Autodesk Inventor part; units mm, degrees
(part 2 of 2)
  spline S117 degree 2 poles (-26.5872, -18.3544) (-26.5872, -19.0932) (-27.8403, -20.0157) (-28.9137, -20.0157) knots 0 0 0 1 2 2 2
  spline S118 degree 2 poles (-28.9137, -20.0157) (-29.5342, -20.0157) (-30.4566, -19.7993) (-30.8607, -19.6279) knots 0 0 0 1 2 2 2
  line L101 (-30.8607, -19.6279) -> (-30.8607, -18.432)
  line L102 (-30.8607, -18.432) -> (-30.7178, -18.432)
  spline S119 degree 2 poles (-30.7178, -18.432) (-30.3219, -18.7504) (-29.3301, -19.0932) (-28.8729, -19.0932) knots 0 0 0 1 2 2 2
  spline S120 degree 2 poles (-28.8729, -19.0932) (-28.7546, -19.0932) (-28.375, -19.0524) (-28.2525, -19.0075) knots 0 0 0 1 2 2 2
  spline S121 degree 2 poles (-28.2525, -19.0075) (-28.1056, -18.9463) (-27.9137, -18.7626) (-27.9137, -18.5871) knots 0 0 0 1 2 2 2
  spline S122 degree 2 poles (-27.9137, -18.5871) (-27.9137, -18.4197) (-28.1913, -18.183) (-28.4607, -18.1177) knots 0 0 0 1 2 2 2
  spline S123 degree 2 poles (-28.4607, -18.1177) (-28.7423, -18.0524) (-29.3709, -17.934) (-29.6484, -17.8442) knots 0 0 0 1 2 2 2
  spline S124 degree 2 poles (-29.6484, -17.8442) (-30.277, -17.6402) (-30.8321, -16.9381) (-30.8321, -16.4157) knots 0 0 0 1 2 2 2
  spline S125 degree 2 poles (-30.8321, -16.4157) (-30.8321, -15.7177) (-29.579, -14.8361) (-28.5954, -14.8361) knots 0 0 0 1 2 2 2
  spline S126 degree 2 poles (-28.5954, -14.8361) (-28.1015, -14.8361) (-27.1382, -15.0279) (-26.7872, -15.1708) knots 0 0 0 1 2 2 2
  line L103 (-26.7872, -15.1708) -> (-26.7872, -16.3218)
  line L104 (-26.7872, -16.3218) -> (-26.926, -16.3218)
  spline S127 degree 2 poles (-26.926, -16.3218) (-27.228, -16.081) (-28.1015, -15.7544) (-28.5586, -15.7544) knots 0 0 0 1 2 2 2
  spline S128 degree 2 poles (-28.5586, -15.7544) (-28.7219, -15.7544) (-29.0403, -15.7993) (-29.1872, -15.8606) knots 0 0 0 1 2 2 2
  spline S129 degree 2 poles (-29.1872, -15.8606) (-29.3178, -15.9095) (-29.5056, -16.1136) (-29.5056, -16.2442) knots 0 0 0 1 2 2 2
  spline S130 degree 2 poles (-29.5056, -16.2442) (-29.5056, -16.4442) (-29.2035, -16.6565) (-28.7831, -16.7422) knots 0 0 0 1 2 2 2
  spline S131 degree 2 poles (-28.7831, -16.7422) (-28.5097, -16.7993) (-27.9995, -16.9055) (-27.7097, -16.9993) knots 0 0 0 1 2 2 2
  spline S132 degree 2 poles (-27.7097, -16.9993) (-27.1342, -17.1912) (-26.5872, -17.8361) (-26.5872, -18.3544) knots 0 0 0 1 2 2 2
  line L105 (-22.0893, -17.2524) -> (-22.0893, -19.9259)
  line L106 (-22.0893, -19.9259) -> (-23.3015, -19.9259)
  line L107 (-23.3015, -19.9259) -> (-23.3015, -18.0402)
  spline S133 degree 2 poles (-23.3015, -18.0402) (-23.3015, -17.7667) (-23.3301, -17.3789) (-23.3872, -17.2606) knots 0 0 0 1 2 2 2
  spline S134 degree 2 poles (-23.3872, -17.2606) (-23.4484, -17.1381) (-23.6933, -17.0279) (-23.9137, -17.0279) knots 0 0 0 1 2 2 2
  spline S135 degree 2 poles (-23.9137, -17.0279) (-24.0933, -17.0279) (-24.428, -17.1708) (-24.5627, -17.2524) knots 0 0 0 1 2 2 2
  line L108 (-24.5627, -17.2524) -> (-24.5627, -19.9259)
  line L109 (-24.5627, -19.9259) -> (-25.775, -19.9259)
  line L110 (-25.775, -19.9259) -> (-25.775, -16.1544)
  line L111 (-25.775, -16.1544) -> (-24.5627, -16.1544)
  line L112 (-24.5627, -16.1544) -> (-24.5627, -16.5708)
  spline S136 degree 2 poles (-24.5627, -16.5708) (-24.2525, -16.3259) (-23.6811, -16.0524) (-23.3342, -16.0524) knots 0 0 0 1 2 2 2
  spline S137 degree 2 poles (-23.3342, -16.0524) (-22.9627, -16.0524) (-22.3954, -16.383) (-22.2321, -16.7055) knots 0 0 0 1 2 2 2
  spline S138 degree 2 poles (-22.2321, -16.7055) (-21.8729, -16.4034) (-21.1872, -16.0524) (-20.8607, -16.0524) knots 0 0 0 1 2 2 2
  spline S139 degree 2 poles (-20.8607, -16.0524) (-20.2484, -16.0524) (-19.6158, -16.783) (-19.6158, -17.4728) knots 0 0 0 1 2 2 2
  line L113 (-19.6158, -17.4728) -> (-19.6158, -19.9259)
  line L114 (-19.6158, -19.9259) -> (-20.828, -19.9259)
  line L115 (-20.828, -19.9259) -> (-20.828, -18.0402)
  spline S140 degree 2 poles (-20.828, -18.0402) (-20.828, -17.7626) (-20.8525, -17.3789) (-20.9137, -17.2606) knots 0 0 0 1 2 2 2
  spline S141 degree 2 poles (-20.9137, -17.2606) (-20.9709, -17.1381) (-21.2158, -17.0279) (-21.4403, -17.0279) knots 0 0 0 1 2 2 2
  spline S142 degree 2 poles (-21.4403, -17.0279) (-21.5913, -17.0279) (-21.8811, -17.13) (-22.0893, -17.2524) knots 0 0 0 1 2 2 2
  spline S143 degree 2 poles (-16.2076, -19.5259) (-16.3056, -19.5993) (-16.5954, -19.8075) (-16.7219, -19.8687) knots 0 0 0 1 2 2 2
  spline S144 degree 2 poles (-16.7219, -19.8687) (-16.9015, -19.9504) (-17.2811, -20.0279) (-17.5097, -20.0279) knots 0 0 0 1 2 2 2
  spline S145 degree 2 poles (-17.5097, -20.0279) (-18.0484, -20.0279) (-18.775, -19.3626) (-18.775, -18.8442) knots 0 0 0 1 2 2 2
  spline S146 degree 2 poles (-18.775, -18.8442) (-18.775, -18.432) (-18.4035, -17.9095) (-18.0648, -17.7585) knots 0 0 0 1 2 2 2
  spline S147 degree 2 poles (-18.0648, -17.7585) (-17.7301, -17.6075) (-16.7342, -17.4769) (-16.1995, -17.4483) knots 0 0 0 1 2 2 2
  line L116 (-16.1995, -17.4483) -> (-16.1995, -17.4279)
  spline S148 degree 2 poles (-16.1995, -17.4279) (-16.1995, -17.1136) (-16.7097, -16.8769) (-17.2076, -16.8769) knots 0 0 0 1 2 2 2
  spline S149 degree 2 poles (-17.2076, -16.8769) (-17.5056, -16.8769) (-18.1872, -17.0891) (-18.3342, -17.1463) knots 0 0 0 1 2 2 2
  line L117 (-18.3342, -17.1463) -> (-18.4444, -17.1463)
  line L118 (-18.4444, -17.1463) -> (-18.4444, -16.2361)
  spline S150 degree 2 poles (-18.4444, -16.2361) (-18.2525, -16.1871) (-17.3913, -16.0483) (-16.9546, -16.0483) knots 0 0 0 1 2 2 2
  spline S151 degree 2 poles (-16.9546, -16.0483) (-15.926, -16.0483) (-15.0076, -16.681) (-15.0076, -17.3626) knots 0 0 0 1 2 2 2
  line L119 (-15.0076, -17.3626) -> (-15.0076, -19.9259)
  line L120 (-15.0076, -19.9259) -> (-16.2076, -19.9259)
  line L121 (-16.2076, -19.9259) -> (-16.2076, -19.5259)
  line L122 (-16.2076, -18.9422) -> (-16.2076, -18.1585)
  spline S152 degree 2 poles (-16.2076, -18.1585) (-16.4525, -18.1789) (-17.0239, -18.2483) (-17.175, -18.2973) knots 0 0 0 1 2 2 2
  spline S153 degree 2 poles (-17.175, -18.2973) (-17.3546, -18.3504) (-17.5464, -18.5708) (-17.5464, -18.7463) knots 0 0 0 1 2 2 2
  spline S154 degree 2 poles (-17.5464, -18.7463) (-17.5464, -18.8646) (-17.5056, -19.0116) (-17.4239, -19.0769) knots 0 0 0 1 2 2 2
  spline S155 degree 2 poles (-17.4239, -19.0769) (-17.3464, -19.1422) (-17.1342, -19.2075) (-16.9056, -19.2075) knots 0 0 0 1 2 2 2
  spline S156 degree 2 poles (-16.9056, -19.2075) (-16.7219, -19.2075) (-16.3505, -19.0606) (-16.2076, -18.9422) knots 0 0 0 1 2 2 2
  line L123 (-11.1627, -17.3055) -> (-11.2688, -17.3055)
  spline S157 degree 2 poles (-11.2688, -17.3055) (-11.3464, -17.2769) (-11.6893, -17.2524) (-11.8035, -17.2524) knots 0 0 0 1 2 2 2
  spline S158 degree 2 poles (-11.8035, -17.2524) (-12.0607, -17.2524) (-12.4566, -17.3177) (-12.6852, -17.3993) knots 0 0 0 1 2 2 2
  line L124 (-12.6852, -17.3993) -> (-12.6852, -19.9259)
  line L125 (-12.6852, -19.9259) -> (-13.8974, -19.9259)
  line L126 (-13.8974, -19.9259) -> (-13.8974, -16.1544)
  line L127 (-13.8974, -16.1544) -> (-12.6852, -16.1544)
  line L128 (-12.6852, -16.1544) -> (-12.6852, -16.7095)
  spline S159 degree 2 poles (-12.6852, -16.7095) (-12.2852, -16.3667) (-11.6974, -16.1422) (-11.4484, -16.1422) knots 0 0 0 1 2 2 2
  spline S160 degree 2 poles (-11.4484, -16.1422) (-11.3831, -16.1422) (-11.2239, -16.1504) (-11.1627, -16.1544) knots 0 0 0 1 2 2 2
  line L129 (-11.1627, -16.1544) -> (-11.1627, -17.3055)
  spline S161 degree 2 poles (-8.0648, -19.8932) (-8.2607, -19.9422) (-8.6974, -19.9993) (-9.0117, -19.9993) knots 0 0 0 1 2 2 2
  spline S162 degree 2 poles (-9.0117, -19.9993) (-9.7178, -19.9993) (-10.4076, -19.4279) (-10.4076, -18.7381) knots 0 0 0 1 2 2 2
  line L130 (-10.4076, -18.7381) -> (-10.4076, -16.9748)
  line L131 (-10.4076, -16.9748) -> (-10.9056, -16.9748)
  line L132 (-10.9056, -16.9748) -> (-10.9056, -16.1544)
  line L133 (-10.9056, -16.1544) -> (-10.4076, -16.1544)
  line L134 (-10.4076, -16.1544) -> (-10.4076, -15.0769)
  line L135 (-10.4076, -15.0769) -> (-9.1954, -15.0769)
  line L136 (-9.1954, -15.0769) -> (-9.1954, -16.1544)
  line L137 (-9.1954, -16.1544) -> (-8.0648, -16.1544)
  line L138 (-8.0648, -16.1544) -> (-8.0648, -16.9748)
  line L139 (-8.0648, -16.9748) -> (-9.1954, -16.9748)
  line L140 (-9.1954, -16.9748) -> (-9.1954, -18.3136)
  spline S163 degree 2 poles (-9.1954, -18.3136) (-9.1954, -18.5095) (-9.1872, -18.8075) (-9.1382, -18.9218) knots 0 0 0 1 2 2 2
  spline S164 degree 2 poles (-9.1382, -18.9218) (-9.0933, -19.0402) (-8.8525, -19.1789) (-8.6239, -19.1789) knots 0 0 0 1 2 2 2
  spline S165 degree 2 poles (-8.6239, -19.1789) (-8.5301, -19.1789) (-8.2239, -19.0973) (-8.1668, -19.0646) knots 0 0 0 1 2 2 2
  line L141 (-8.1668, -19.0646) -> (-8.0648, -19.0646)
  line L142 (-8.0648, -19.0646) -> (-8.0648, -19.8932)
  spline S166 degree 2 poles (-0.0648, -17.4279) (-0.0648, -18.6238) (-1.4321, -20.032) (-2.6403, -20.032) knots 0 0 0 1 2 2 2
  spline S167 degree 2 poles (-2.6403, -20.032) (-3.8484, -20.032) (-5.2158, -18.6238) (-5.2158, -17.4279) knots 0 0 0 1 2 2 2
  spline S168 degree 2 poles (-5.2158, -17.4279) (-5.2158, -16.2197) (-3.8484, -14.8197) (-2.6403, -14.8197) knots 0 0 0 1 2 2 2
  spline S169 degree 2 poles (-2.6403, -14.8197) (-1.4403, -14.8197) (-0.0648, -16.2197) (-0.0648, -17.4279) knots 0 0 0 1 2 2 2
  spline S170 degree 2 poles (-1.7709, -18.6973) (-1.5831, -18.4687) (-1.4035, -17.8442) (-1.4035, -17.4238) knots 0 0 0 1 2 2 2
  spline S171 degree 2 poles (-1.4035, -17.4238) (-1.4035, -16.9748) (-1.6117, -16.3422) (-1.779, -16.1463) knots 0 0 0 1 2 2 2
  spline S172 degree 2 poles (-1.779, -16.1463) (-1.9505, -15.9422) (-2.3954, -15.7626) (-2.6403, -15.7626) knots 0 0 0 1 2 2 2
  spline S173 degree 2 poles (-2.6403, -15.7626) (-2.8852, -15.7626) (-3.3178, -15.9381) (-3.4974, -16.1381) knots 0 0 0 1 2 2 2
  spline S174 degree 2 poles (-3.4974, -16.1381) (-3.6648, -16.3259) (-3.877, -16.9912) (-3.877, -17.4279) knots 0 0 0 1 2 2 2
  spline S175 degree 2 poles (-3.877, -17.4279) (-3.877, -17.8769) (-3.6729, -18.5055) (-3.5056, -18.7014) knots 0 0 0 1 2 2 2
  spline S176 degree 2 poles (-3.5056, -18.7014) (-3.3382, -18.9014) (-2.8852, -19.0891) (-2.6403, -19.0891) knots 0 0 0 1 2 2 2
  spline S177 degree 2 poles (-2.6403, -19.0891) (-2.3913, -19.0891) (-1.9423, -18.8973) (-1.7709, -18.6973) knots 0 0 0 1 2 2 2
  spline S178 degree 2 poles (4.7883, -17.9871) (4.7883, -18.4565) (4.5026, -19.2197) (4.274, -19.4687) knots 0 0 0 1 2 2 2
  spline S179 degree 2 poles (4.274, -19.4687) (4.0291, -19.73) (3.421, -19.9993) (3.0699, -19.9993) knots 0 0 0 1 2 2 2
  spline S180 degree 2 poles (3.0699, -19.9993) (2.7516, -19.9993) (2.3026, -19.8606) (2.0658, -19.7381) knots 0 0 0 1 2 2 2
  line L143 (2.0658, -19.7381) -> (2.0658, -21.3095)
  line L144 (2.0658, -21.3095) -> (0.8536, -21.3095)
  line L145 (0.8536, -21.3095) -> (0.8536, -16.1544)
  line L146 (0.8536, -16.1544) -> (2.0658, -16.1544)
  line L147 (2.0658, -16.1544) -> (2.0658, -16.5463)
  spline S181 degree 2 poles (2.0658, -16.5463) (2.3434, -16.3259) (2.923, -16.0524) (3.3026, -16.0524) knots 0 0 0 1 2 2 2
  spline S182 degree 2 poles (3.3026, -16.0524) (4.0087, -16.0524) (4.7883, -17.0851) (4.7883, -17.9871) knots 0 0 0 1 2 2 2
  spline S183 degree 2 poles (3.5434, -18.0157) (3.5434, -17.4646) (3.1679, -16.9708) (2.7638, -16.9708) knots 0 0 0 1 2 2 2
  spline S184 degree 2 poles (2.7638, -16.9708) (2.5924, -16.9708) (2.2291, -17.0728) (2.0658, -17.1708) knots 0 0 0 1 2 2 2
  line L148 (2.0658, -17.1708) -> (2.0658, -19.0646)
  spline S185 degree 2 poles (2.0658, -19.0646) (2.1883, -19.1095) (2.4618, -19.1381) (2.5965, -19.1381) knots 0 0 0 1 2 2 2
  spline S186 degree 2 poles (2.5965, -19.1381) (3.074, -19.1381) (3.5434, -18.5789) (3.5434, -18.0157) knots 0 0 0 1 2 2 2
  line L149 (9.3761, -18.2646) -> (6.6046, -18.2646)
  spline S187 degree 2 poles (6.6046, -18.2646) (6.6332, -18.7095) (7.2536, -19.1789) (7.8618, -19.1789) knots 0 0 0 1 2 2 2
  spline S188 degree 2 poles (7.8618, -19.1789) (8.2414, -19.1789) (8.9638, -18.9055) (9.172, -18.7463) knots 0 0 0 1 2 2 2
  line L150 (9.172, -18.7463) -> (9.3067, -18.7463)
  line L151 (9.3067, -18.7463) -> (9.3067, -19.7177)
  spline S189 degree 2 poles (9.3067, -19.7177) (8.8985, -19.881) (8.172, -20.0279) (7.7312, -20.0279) knots 0 0 0 1 2 2 2
  spline S190 degree 2 poles (7.7312, -20.0279) (6.5924, -20.0279) (5.3842, -19.0075) (5.3842, -18.0606) knots 0 0 0 1 2 2 2
  spline S191 degree 2 poles (5.3842, -18.0606) (5.3842, -17.13) (6.5312, -16.0361) (7.5271, -16.0361) knots 0 0 0 1 2 2 2
  spline S192 degree 2 poles (7.5271, -16.0361) (8.4495, -16.0361) (9.3761, -16.9667) (9.3761, -17.8402) knots 0 0 0 1 2 2 2
  line L152 (9.3761, -17.8402) -> (9.3761, -18.2646)
  spline S193 degree 2 poles (8.172, -17.5544) (8.1638, -17.1748) (7.8046, -16.7912) (7.4291, -16.7912) knots 0 0 0 1 2 2 2
  spline S194 degree 2 poles (7.4291, -16.7912) (7.0781, -16.7912) (6.6291, -17.1544) (6.6005, -17.5544) knots 0 0 0 1 2 2 2
  line L153 (6.6005, -17.5544) -> (8.172, -17.5544)
  line L154 (14.0169, -19.9259) -> (12.8046, -19.9259)
  line L155 (12.8046, -19.9259) -> (12.8046, -18.0565)
  spline S195 degree 2 poles (12.8046, -18.0565) (12.8046, -17.8279) (12.7556, -17.3748) (12.7026, -17.2646) knots 0 0 0 1 2 2 2
  spline S196 degree 2 poles (12.7026, -17.2646) (12.6332, -17.1422) (12.3761, -17.0279) (12.1434, -17.0279) knots 0 0 0 1 2 2 2
  spline S197 degree 2 poles (12.1434, -17.0279) (11.9801, -17.0279) (11.6414, -17.134) (11.4414, -17.2524) knots 0 0 0 1 2 2 2
  line L156 (11.4414, -17.2524) -> (11.4414, -19.9259)
  line L157 (11.4414, -19.9259) -> (10.2291, -19.9259)
  line L158 (10.2291, -19.9259) -> (10.2291, -16.1544)
  line L159 (10.2291, -16.1544) -> (11.4414, -16.1544)
  line L160 (11.4414, -16.1544) -> (11.4414, -16.5708)
  spline S198 degree 2 poles (11.4414, -16.5708) (11.7638, -16.3218) (12.3556, -16.0524) (12.7189, -16.0524) knots 0 0 0 1 2 2 2
  spline S199 degree 2 poles (12.7189, -16.0524) (13.3312, -16.0524) (14.0169, -16.7626) (14.0169, -17.4728) knots 0 0 0 1 2 2 2
  line L161 (14.0169, -17.4728) -> (14.0169, -19.9259)
  line L162 (21.1516, -19.9259) -> (17.5434, -19.9259)
  line L163 (17.5434, -19.9259) -> (17.5434, -14.9259)
  line L164 (17.5434, -14.9259) -> (18.8332, -14.9259)
  line L165 (18.8332, -14.9259) -> (18.8332, -18.9585)
  line L166 (18.8332, -18.9585) -> (21.1516, -18.9585)
  line L167 (21.1516, -18.9585) -> (21.1516, -19.9259)
  spline S200 degree 2 poles (24.1475, -19.5259) (24.0495, -19.5993) (23.7597, -19.8075) (23.6332, -19.8687) knots 0 0 0 1 2 2 2
  spline S201 degree 2 poles (23.6332, -19.8687) (23.4536, -19.9504) (23.074, -20.0279) (22.8454, -20.0279) knots 0 0 0 1 2 2 2
  spline S202 degree 2 poles (22.8454, -20.0279) (22.3067, -20.0279) (21.5801, -19.3626) (21.5801, -18.8442) knots 0 0 0 1 2 2 2
  spline S203 degree 2 poles (21.5801, -18.8442) (21.5801, -18.432) (21.9516, -17.9095) (22.2903, -17.7585) knots 0 0 0 1 2 2 2
  spline S204 degree 2 poles (22.2903, -17.7585) (22.625, -17.6075) (23.621, -17.4769) (24.1556, -17.4483) knots 0 0 0 1 2 2 2
  line L168 (24.1556, -17.4483) -> (24.1556, -17.4279)
  spline S205 degree 2 poles (24.1556, -17.4279) (24.1556, -17.1136) (23.6454, -16.8769) (23.1475, -16.8769) knots 0 0 0 1 2 2 2
  spline S206 degree 2 poles (23.1475, -16.8769) (22.8495, -16.8769) (22.1679, -17.0891) (22.021, -17.1463) knots 0 0 0 1 2 2 2
  line L169 (22.021, -17.1463) -> (21.9107, -17.1463)
  line L170 (21.9107, -17.1463) -> (21.9107, -16.2361)
  spline S207 degree 2 poles (21.9107, -16.2361) (22.1026, -16.1871) (22.9638, -16.0483) (23.4005, -16.0483) knots 0 0 0 1 2 2 2
  spline S208 degree 2 poles (23.4005, -16.0483) (24.4291, -16.0483) (25.3475, -16.681) (25.3475, -17.3626) knots 0 0 0 1 2 2 2
  line L171 (25.3475, -17.3626) -> (25.3475, -19.9259)
  line L172 (25.3475, -19.9259) -> (24.1475, -19.9259)
  line L173 (24.1475, -19.9259) -> (24.1475, -19.5259)
  line L174 (24.1475, -18.9422) -> (24.1475, -18.1585)
  spline S209 degree 2 poles (24.1475, -18.1585) (23.9026, -18.1789) (23.3312, -18.2483) (23.1801, -18.2973) knots 0 0 0 1 2 2 2
  spline S210 degree 2 poles (23.1801, -18.2973) (23.0005, -18.3504) (22.8087, -18.5708) (22.8087, -18.7463) knots 0 0 0 1 2 2 2
  spline S211 degree 2 poles (22.8087, -18.7463) (22.8087, -18.8646) (22.8495, -19.0116) (22.9312, -19.0769) knots 0 0 0 1 2 2 2
  spline S212 degree 2 poles (22.9312, -19.0769) (23.0087, -19.1422) (23.221, -19.2075) (23.4495, -19.2075) knots 0 0 0 1 2 2 2
  spline S213 degree 2 poles (23.4495, -19.2075) (23.6332, -19.2075) (24.0046, -19.0606) (24.1475, -18.9422) knots 0 0 0 1 2 2 2
  spline S214 degree 2 poles (30.3924, -17.9871) (30.3924, -18.8769) (29.4087, -19.9993) (28.674, -19.9993) knots 0 0 0 1 2 2 2
  spline S215 degree 2 poles (28.674, -19.9993) (28.3597, -19.9993) (27.8863, -19.8646) (27.6699, -19.7381) knots 0 0 0 1 2 2 2
  line L175 (27.6699, -19.7381) -> (27.621, -19.9259)
  line L176 (27.621, -19.9259) -> (26.4577, -19.9259)
  line L177 (26.4577, -19.9259) -> (26.4577, -14.7014)
  line L178 (26.4577, -14.7014) -> (27.6699, -14.7014)
  line L179 (27.6699, -14.7014) -> (27.6699, -16.5504)
  spline S216 degree 2 poles (27.6699, -16.5504) (27.9475, -16.3259) (28.5271, -16.0524) (28.9067, -16.0524) knots 0 0 0 1 2 2 2
  spline S217 degree 2 poles (28.9067, -16.0524) (29.621, -16.0524) (30.3924, -17.081) (30.3924, -17.9871) knots 0 0 0 1 2 2 2
  spline S218 degree 2 poles (29.1475, -18.0157) (29.1475, -17.5136) (28.8046, -16.9708) (28.3679, -16.9708) knots 0 0 0 1 2 2 2
  spline S219 degree 2 poles (28.3679, -16.9708) (28.1965, -16.9708) (27.8332, -17.0728) (27.6699, -17.1708) knots 0 0 0 1 2 2 2
  line L180 (27.6699, -17.1708) -> (27.6699, -19.0565)
  spline S220 degree 2 poles (27.6699, -19.0565) (27.8005, -19.1055) (28.0332, -19.1381) (28.2005, -19.1381) knots 0 0 0 1 2 2 2
  spline S221 degree 2 poles (28.2005, -19.1381) (28.6781, -19.1381) (29.1475, -18.5748) (29.1475, -18.0157) knots 0 0 0 1 2 2 2
  point P0 (0, 0)
  constraints: 2 other
extrude "Extrusion30" cut sketch "Sketch38" against normal blind 2.5 bodies 6
ref_plane "Work Plane7" through (0, -75, 15.7021) normal (0, 0, 1) x (1, 0, 0)
extrude "Extrusion31" cut sketch "Sketch10" along normal mid plane 26 contours A2 | A3 bodies 1
mirror "Mirror4" about plane through (0, 0, 0) normal (1, 0, 0) of "Extrusion8", "Extrusion31", "Extrusion9" bodies 1
sketch "Sketch41" plane through (0, 0, -2.5) normal (0, 0, -1) x (-1, 0, 0)
  circle A0 centre (-41.19, -41.4743) radius 1.25 projected
  circle A1 centre (-42, -63) radius 1.15 projected
  circle A2 centre (41.19, -41.4743) radius 1.25 projected
  circle A3 centre (42, -63) radius 1.15 projected
  point P0 (0, 0)
hole "Hole1" at (42, -63, -2.5) at (41.19, -41.4743, -2.5) at (-42, -63, -2.5) at (-41.19, -41.4743, -2.5) direction (0, 0, 1) diameter 2.5 end through all counterbore diameter 4.5 counterbore depth 2.5 bodies 1
sketch "Sketch42" plane through (-40, 75, 22.5) normal (0, 1, 0) x (1, 0, 0)
  line L0 (80, 0) -> (0, 0) projected
  line L1 (0, 0) -> (80, 0) projected
  line L2 (40, 0) -> (40, 25)
  line L3 (80, 25) -> (0, 25) projected
  line L4 (32, 8) -> (48, 8)
  line L5 (48, 8) -> (48, 16)
  line L6 (48, 16) -> (32, 16)
  line L7 (32, 16) -> (32, 8)
  line L8 (40, 32.0957) -> (40, -17.5741) projected
  point P0 (40, 22.5)
  dimension "d181" = 16
  dimension "d182" = 8
  dimension "d183" = 8
  constraints: 10 end point, 2 midpoint, 2 parallel, 1 horizontal, 1 perpendicular, 1 other
  measures "d181" distance of L6.end L5.end
  measures "d182" distance of L5.end L4.end
  measures "d183" distance between parallel lines of L0 L4
extrude "Extrusion32" cut sketch "Sketch42" against normal up to next bodies 1
equation "\"d7\" = radio_esquina_base"
equation "\"d8\" = radio_esquina_base"
equation "\"d9\" = radio_esquina_base"
equation "\"d30\" = d25"
equation "\"d39\" = -0.5 * largo_galga"
